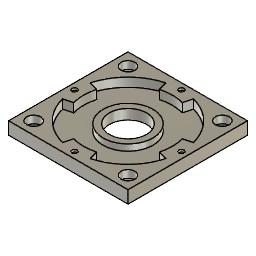
OpenATC-Assembly (Autodesk Fusion 360 archive; units mm, degrees)
design "OpenATC-Base-holder"
Autodesk Fusion 360 part; units mm, degrees
note: some values were not read from the file. Chosen so that the rebuilt part matches the saved one: a direction; a side.
sketch "Sketch1" plane through (0, 0, 0) normal (0, 0, 1) x (1, 0, 0)
  line L0 (-47.5, -47.5) -> (47.5, -47.5)
  line L1 (47.5, -47.5) -> (47.5, 47.5)
  line L2 (47.5, 47.5) -> (-47.5, 47.5)
  line L3 (-47.5, 47.5) -> (-47.5, -47.5)
  line L4 (-37.5, 37.5) -> (-37.5, -37.5) construction
  line L5 (-37.5, -37.5) -> (37.5, -37.5) construction
  line L6 (37.5, 37.5) -> (37.5, -37.5) construction
  line L7 (-37.5, 37.5) -> (-24.7362, 37.5)
  line L8 (-24.7362, 37.5) -> (37.5, 37.5) construction
  line L9 (-47.5, 47.5) -> (47.5, -47.5) construction
  line L10 (-47.5, -47.5) -> (47.5, 47.5) construction
  point P0 (-37.5, 37.5)
  point P1 (37.5, 37.5)
  point P2 (-37.5, -37.5)
  point P3 (37.5, -37.5)
  dimension "d33" = 10
  dimension "d34" = 75
  dimension "d35" = 75
  constraint horizontal L0
  constraint vertical L1
  constraint horizontal L2
  constraint vertical L3
  constraint coincident P0 L4.start
  constraint coincident P2 L4.end
  constraint coincident P3 L5.end
  constraint horizontal L5
  constraint coincident P1 L6.start
  constraint perpendicular L4 L7
  constraint vertical L6
  constraint vertical L4
  constraint horizontal L8
  constraint coincident origin L10
  constraint coincident origin L9
  constraint coincident L0.start L3.end
  constraint coincident P2 L10
  constraint coincident P0 L9
  constraint coincident P1 L10
  measures "d33" distance of L1 L6
  measures "d34" distance of P2 P3
  measures "d35" distance of P0 P2
extrude "Extrude1" add sketch "Sketch1" along normal blind 10
sketch "Sketch2" plane through (0, 0, 10) normal (0, 0, 1) x (-1, 0, 0)
  line L0 (47.5, -47.5) -> (47.5, 47.5)
  line L1 (47.5, 47.5) -> (-47.5, 47.5)
  line L2 (-47.5, 47.5) -> (-47.5, -47.5)
  line L3 (-47.5, -47.5) -> (47.5, -47.5)
  circle A0 centre (0, 0) radius 19.8
  circle A1 centre (0, 0) radius 42.5
  line L4 (0, 0) -> (0, -42.5) construction
  line L5 (10.9998, -41.0518) -> (9.1234, -34.0489)
  line L6 (0, 0) -> (9.1234, -34.0489) construction
  line L7 (0, 0) -> (-9.1234, -34.0489) construction
  line L8 (-9.1234, -34.0489) -> (-10.9998, -41.0518)
  arc A2 (-9.1234, -34.0489) -> (9.1234, -34.0489) centre (0, 0) ccw
  line L9 (41.0518, 10.9998) -> (34.0489, 9.1234)
  arc A3 (34.0489, -9.1234) -> (34.0489, 9.1234) centre (0, 0) ccw
  line L10 (34.0489, -9.1234) -> (41.0518, -10.9998)
  line L11 (-10.9998, 41.0518) -> (-9.1234, 34.0489)
  arc A4 (9.1234, 34.0489) -> (-9.1234, 34.0489) centre (0, 0) ccw
  line L12 (9.1234, 34.0489) -> (10.9998, 41.0518)
  line L13 (-41.0518, -10.9998) -> (-34.0489, -9.1234)
  arc A5 (-34.0489, 9.1234) -> (-34.0489, -9.1234) centre (0, 0) ccw
  line L14 (-34.0489, 9.1234) -> (-41.0518, 10.9998)
  dimension "d9" = 39.6
  dimension "d10" = 85
  dimension "d11" = 35.25
  dimension "d12" = 15
  dimension "d13" = 15
  dimension "d15" = 360
  constraint coincident A0.centre A1.centre
  constraint coincident A1 L4.end
  constraint vertical L4
  constraint coincident A1 L5.start
  constraint coincident A1 L8.end
  constraint parallel L7 L8
  constraint parallel L5 L6
  constraint concentric A1 A2
  measures "d9" diameter of A0
  measures "d10" diameter of A1
  measures "d11" radius of A2
  measures "d12" angle of L4 L5
  measures "d13" angle of L4 L7
extrude "Extrude2" cut sketch "Sketch2" against normal blind 7 contours A1 L5 L8 A2 L9 A3 L10 L11 A4 L12 L13 A5 L14
sketch "Sketch3" plane through (0, 0, 10) normal (0, 0, 1) x (-1, 0, 0)
  circle A0 centre (0, 0) radius 19.8
extrude "Extrude3" cut sketch "Sketch3" against normal up to surface (2 mm away)
sketch "Sketch4" plane through (0, 0, 8) normal (0, 0, 1) x (-1, 0, 0)
  circle A0 centre (0, 0) radius 19.8
  circle A1 centre (0, 0) radius 14.8
  dimension "d36" = 5
  constraint concentric A0 A1
  measures "d36" distance of A0 A1
extrude "Extrude4" cut sketch "Sketch4" against normal through all contours A1
sketch "Sketch6" plane through (0, 0, 10) normal (0, 0, 1) x (-1, 0, 0)
  line L0 (47.5, -47.5) -> (47.5, 47.5)
  line L1 (47.5, 47.5) -> (-47.5, 47.5)
  line L2 (-47.5, 47.5) -> (-47.5, -47.5)
  line L3 (-47.5, -47.5) -> (47.5, -47.5)
  arc A0 (-10.9998, 41.0518) -> (-41.0518, 10.9998) centre (0, 0) ccw
  line L4 (-10.9998, 41.0518) -> (-9.1234, 34.0489)
  arc A1 (9.1234, 34.0489) -> (-9.1234, 34.0489) centre (0, 0) ccw
  line L5 (9.1234, 34.0489) -> (10.9998, 41.0518)
  arc A2 (41.0518, 10.9998) -> (10.9998, 41.0518) centre (0, 0) ccw
  line L6 (41.0518, 10.9998) -> (34.0489, 9.1234)
  arc A3 (34.0489, -9.1234) -> (34.0489, 9.1234) centre (0, 0) ccw
  line L7 (34.0489, -9.1234) -> (41.0518, -10.9998)
  arc A4 (10.9998, -41.0518) -> (41.0518, -10.9998) centre (0, 0) ccw
  line L8 (37.5, -37.5) -> (-37.5, -37.5) construction
  line L9 (-37.5, -37.5) -> (-37.5, 37.5) construction
  line L10 (-37.5, 37.5) -> (37.5, 37.5) construction
  line L11 (37.5, 37.5) -> (37.5, -37.5) construction
  line L12 (-9.1234, -34.0489) -> (-10.9998, -41.0518)
  arc A5 (-41.0518, -10.9998) -> (-10.9998, -41.0518) centre (0, 0) ccw
  line L13 (-41.0518, -10.9998) -> (-34.0489, -9.1234)
  arc A6 (-34.0489, 9.1234) -> (-34.0489, -9.1234) centre (0, 0) ccw
  line L14 (-34.0489, 9.1234) -> (-41.0518, 10.9998)
  line L15 (10.9998, -41.0518) -> (9.1234, -34.0489)
  arc A7 (-9.1234, -34.0489) -> (9.1234, -34.0489) centre (0, 0) ccw
  point P0 (37.5, -37.5)
  point P1 (-37.5, -37.5)
  point P2 (-37.5, 37.5)
  point P3 (37.5, 37.5)
  dimension "d22" = 10
  dimension "d23" = 10
  dimension "d24" = 10
  dimension "d25" = 10
  constraint coincident P0 L8.start
  constraint coincident P1 L8.end
  constraint parallel L3 L8
  constraint coincident P2 L9.end
  constraint perpendicular L3 L9
  constraint coincident P3 L10.end
  constraint perpendicular L9 L10
  constraint vertical L11
  measures "d22" distance of L1 L10
  measures "d23" distance of L0 L11
  measures "d24" distance of L3 L8
  measures "d25" distance of L2 L9
hole "Hole1" at (-37.5, -37.5, 10) at (-37.5, 37.5, 10) at (37.5, 37.5, 10) at (37.5, -37.5, 10) direction (0, 0, -1) diameter 6.6 end through all counterbore diameter 11 counterbore depth 6
sketch "Sketch7" plane through (0, 0, 10) normal (0, 0, 1) x (-1, 0, 0)
  circle A0 centre (-37.5, -37.5) radius 5.5
  circle A1 centre (37.5, 37.5) radius 5.5
  circle A2 centre (37.5, -37.5) radius 5.5
  circle A3 centre (-37.5, 37.5) radius 5.5
  line L0 (47.5, -47.5) -> (47.5, 47.5)
  line L1 (47.5, 47.5) -> (-47.5, 47.5)
  line L2 (-47.5, 47.5) -> (-47.5, -47.5)
  line L3 (-47.5, -47.5) -> (47.5, -47.5)
  line L4 (-9.1234, -34.0489) -> (-10.9998, -41.0518)
  arc A4 (-41.0518, -10.9998) -> (-10.9998, -41.0518) centre (0, 0) ccw
  line L5 (-41.0518, -10.9998) -> (-34.0489, -9.1234)
  arc A5 (-34.0489, 9.1234) -> (-34.0489, -9.1234) centre (0, 0) ccw
  line L6 (-34.0489, 9.1234) -> (-41.0518, 10.9998)
  arc A6 (-10.9998, 41.0518) -> (-41.0518, 10.9998) centre (0, 0) ccw
  line L7 (-10.9998, 41.0518) -> (-9.1234, 34.0489)
  arc A7 (9.1234, 34.0489) -> (-9.1234, 34.0489) centre (0, 0) ccw
  line L8 (9.1234, 34.0489) -> (10.9998, 41.0518)
  arc A8 (41.0518, 10.9998) -> (10.9998, 41.0518) centre (0, 0) ccw
  line L9 (41.0518, 10.9998) -> (34.0489, 9.1234)
  arc A9 (34.0489, -9.1234) -> (34.0489, 9.1234) centre (0, 0) ccw
  line L10 (34.0489, -9.1234) -> (41.0518, -10.9998)
  arc A10 (10.9998, -41.0518) -> (41.0518, -10.9998) centre (0, 0) ccw
  line L11 (10.9998, -41.0518) -> (9.1234, -34.0489)
  arc A11 (-9.1234, -34.0489) -> (9.1234, -34.0489) centre (0, 0) ccw
  line L12 (47.5, 0) -> (-47.5, 0) construction
  line L13 (0, -47.5) -> (0, 47.5) construction
  point P0 (42.5, 0)
  point P1 (-42.5, 0)
  point P2 (0, -42.5)
  point P3 (0, 42.5)
  dimension "d37" = 5
  dimension "d38" = 5
  dimension "d39" = 5
  dimension "d40" = 5
  constraint midpoint L0 L12.start
  constraint midpoint L2 L12.end
  constraint midpoint L3 L13.start
  constraint midpoint L1 L13.end
  constraint coincident L12 P0
  constraint coincident L12 P1
  constraint coincident L13 P2
  constraint coincident L13 P3
  measures "d37" distance of L0 P0
  measures "d38" distance of L1 P3
  measures "d39" distance of L2 P1
  measures "d40" distance of L3 P2
hole "Hole2" at (0, 42.5, 10) at (-42.5, 0, 10) at (0, -42.5, 10) at (42.5, 0, 10) direction (0, 0, -1) diameter 3.332 end through all
thread "Thread1" "ISO Metric profile 4.0 M4x0.7 M4x0.7 6H" thread offset 0 thread depth 7.4
chamfer "Chamfer1" distance 0.4 angle 75 4 edges at (-1.5533, 43.1025, 10) (40.9467, 0.6025, 10) (-1.5533, -41.8975, 10) (-44.0533, 0.6025, 10) measured on face at (-5.2099, -39.359, 10) measured on face at (-5.2099, -39.359, 10) measured on face at (-5.2099, -39.359, 10) measured on face at (-5.2099, -39.359, 10)
equation "d13 = d12"
equation "d23 = d22"
equation "d24 = d22"
equation "d25 = d22"
equation "d35 = d34"
equation "d38 = d37"
equation "d39 = d37"
equation "d40 = d37"

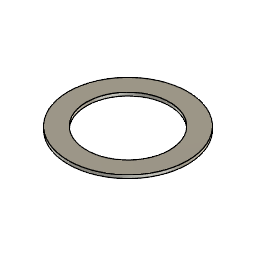
design "Washer-ID_25mm-OD_36mm"
Autodesk Fusion 360 part; units mm, degrees
sketch "Sketch1" plane through (0, 0, 0) normal (0, 0, 1) x (1, 0, 0)
  circle A0 centre (0, 0) radius 12.5
  circle A1 centre (0, 0) radius 18
  dimension "d1" = 25
  dimension "d2" = 36
  constraint coincident A0.centre A1.centre
  constraint concentric A0 A1
  measures "d1" diameter of A0
  measures "d2" diameter of A1
extrude "Extrude1" add sketch "Sketch1" along normal blind 1

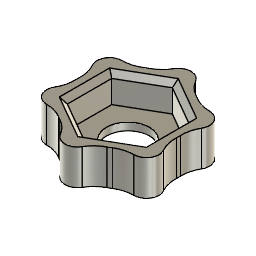
design "OpenATC-ER20-A-Nut-holder"
Autodesk Fusion 360 part; units mm, degrees
sketch "Sketch1" plane through (0, 0, 0) normal (0, 0, 1) x (1, 0, 0)
  circle A0 centre (0, 0) radius 8.5
  circle A1 centre (0, 0) radius 20
  dimension "d1" = 17
  dimension "d2" = 40
  constraint coincident A0.centre A1.centre
  measures "d1" diameter of A0
  measures "d2" diameter of A1
extrude "Extrude1" add sketch "Sketch1" along normal blind 14
sketch "Sketch2" plane through (0, 0, 14) normal (0, 0, 1) x (-1, 0, 0)
  circle A0 centre (0, 0) radius 8.5
  circle A1 centre (0, 0) radius 20
  line L0 (-15.25, -8.8046) -> (0, -17.6092)
  line L1 (0, -17.6092) -> (15.25, -8.8046)
  line L2 (15.25, -8.8046) -> (15.25, 8.8046)
  line L3 (15.25, 8.8046) -> (0, 17.6092)
  line L4 (0, 17.6092) -> (-15.25, 8.8046)
  line L5 (-15.25, 8.8046) -> (-15.25, -8.8046)
  line L6 (0, 0) -> (0, -24.7489) construction
  dimension "d5" = 15.25
  constraint coincident A0.centre A1.centre
  constraint vertical L6
  constraint coincident L0.end L6
  measures "d5" distance of A0.centre L5
extrude "Extrude2" cut sketch "Sketch2" against normal blind 11 contours L0 L1 L2 L3 L4 L5
sketch "Sketch3" plane through (0, 0, 14) normal (0, 0, 1) x (-1, 0, 0)
  line L0 (0, -17.6092) -> (-15.25, -8.8046)
  line L1 (-15.25, -8.8046) -> (-15.25, 8.8046)
  line L2 (-15.25, 8.8046) -> (0, 17.6092)
  line L3 (0, 17.6092) -> (15.25, 8.8046)
  line L4 (15.25, 8.8046) -> (15.25, -8.8046)
  line L5 (15.25, -8.8046) -> (0, -17.6092)
  circle A0 centre (0, 0) radius 20
  line L6 (0, -20) -> (0, 20) construction
  line L7 (20, 0) -> (-20, 0) construction
  arc A1 (-4.3301, -22.5) -> (4.3301, -22.5) centre (0, -20) ccw
  line L8 (0, -20) -> (0, -25) construction
  line L9 (0, -20) -> (4.3301, -22.5) construction
  line L10 (0, -20) -> (-4.3301, -22.5) construction
  arc A2 (9.3264, -17.6923) -> (4.3301, -22.5) centre (15.1554, -28.75) ccw
  arc A3 (-4.3301, -22.5) -> (-9.3264, -17.6923) centre (-15.1554, -28.75) ccw
  arc A4 (-9.3264, -17.6923) -> (9.3264, -17.6923) centre (0, 0) ccw
  arc A5 (17.3205, -15) -> (21.6506, -7.5) centre (17.3205, -10) ccw
  arc A6 (17.3205, -15) -> (10.6588, -16.9231) centre (17.3205, -27.5) ccw
  arc A7 (10.6588, -16.9231) -> (19.9852, -0.7692) centre (0, 0) ccw
  arc A8 (19.9852, -0.7692) -> (21.6506, -7.5) centre (32.476, -1.25) ccw
  arc A9 (21.6506, 7.5) -> (17.3205, 15) centre (17.3205, 10) ccw
  arc A10 (21.6506, 7.5) -> (19.9852, 0.7692) centre (32.476, 1.25) ccw
  arc A11 (19.9852, 0.7692) -> (10.6588, 16.9231) centre (0, 0) ccw
  arc A12 (10.6588, 16.9231) -> (17.3205, 15) centre (17.3205, 27.5) ccw
  arc A13 (4.3301, 22.5) -> (-4.3301, 22.5) centre (0, 20) ccw
  arc A14 (4.3301, 22.5) -> (9.3264, 17.6923) centre (15.1554, 28.75) ccw
  arc A15 (9.3264, 17.6923) -> (-9.3264, 17.6923) centre (0, 0) ccw
  arc A16 (-9.3264, 17.6923) -> (-4.3301, 22.5) centre (-15.1554, 28.75) ccw
  arc A17 (-17.3205, 15) -> (-21.6506, 7.5) centre (-17.3205, 10) ccw
  arc A18 (-17.3205, 15) -> (-10.6588, 16.9231) centre (-17.3205, 27.5) ccw
  arc A19 (-10.6588, 16.9231) -> (-19.9852, 0.7692) centre (0, 0) ccw
  arc A20 (-19.9852, 0.7692) -> (-21.6506, 7.5) centre (-32.476, 1.25) ccw
  arc A21 (-21.6506, -7.5) -> (-17.3205, -15) centre (-17.3205, -10) ccw
  arc A22 (-21.6506, -7.5) -> (-19.9852, -0.7692) centre (-32.476, -1.25) ccw
  arc A23 (-19.9852, -0.7692) -> (-10.6588, -16.9231) centre (0, 0) ccw
  arc A24 (-10.6588, -16.9231) -> (-17.3205, -15) centre (-17.3205, -27.5) ccw
  dimension "d10" = 60
  dimension "d11" = 60
  dimension "d12" = 5
  dimension "d14" = 360
  constraint coincident A0 L6.start
  constraint coincident A0 L6.end
  constraint vertical L6
  constraint coincident A0 L7.start
  constraint coincident A0 L7.end
  constraint perpendicular L6 L7
  constraint coincident A0.centre L6
  constraint coincident A0.centre L7
  constraint parallel L6 L8
  constraint coincident L6.start A1.centre
  constraint tangent A0 A2
  constraint coincident A0 A2.start
  constraint tangent A1 A2
  constraint tangent A0 A3
  constraint coincident A0 A3.end
  constraint tangent A1 A3
  constraint coincident A1 L8.end
  constraint coincident L6.start A4
  measures "d10" angle of L8 L10
  measures "d11" angle of L8 L9
  measures "d12" radius of A1
extrude "Extrude3" add sketch "Sketch3" against normal up to surface (14 mm away) contours A0 A9 A10 A11 A12 | A0 A5 A6 A7 A8 | A0 A13 A14 A15 A16 | A0 A1 A2 A3 A4 | A0 A17 A18 A19 A20 | A0 A21 A22 A23 A24
chamfer "Chamfer1" distance 2 angle 45 6 edges at (-7.625, 13.2069, 14) (-15.25, 0, 14) (-7.625, -13.2069, 14) (7.625, -13.2069, 14) (15.25, 0, 14) (7.625, 13.2069, 14)
sketch "Sketch4" plane through (0, 0, 0) normal (0, 0, -1) x (1, 0, 0)
  circle A0 centre (0, 0) radius 8.5
  arc A1 (-9.3264, 17.6923) -> (-10.6588, 16.9231) centre (0, 0) ccw
  arc A2 (-17.3205, 15) -> (-10.6588, 16.9231) centre (-17.3205, 27.5) ccw
  arc A3 (-17.3205, 15) -> (-21.6506, 7.5) centre (-17.3205, 10) ccw
  arc A4 (-19.9852, 0.7692) -> (-21.6506, 7.5) centre (-32.476, 1.25) ccw
  arc A5 (-19.9852, 0.7692) -> (-19.9852, -0.7692) centre (0, 0) ccw
  arc A6 (-21.6506, -7.5) -> (-19.9852, -0.7692) centre (-32.476, -1.25) ccw
  arc A7 (-21.6506, -7.5) -> (-17.3205, -15) centre (-17.3205, -10) ccw
  arc A8 (-10.6588, -16.9231) -> (-17.3205, -15) centre (-17.3205, -27.5) ccw
  arc A9 (-10.6588, -16.9231) -> (-9.3264, -17.6923) centre (0, 0) ccw
  arc A10 (-4.3301, -22.5) -> (-9.3264, -17.6923) centre (-15.1554, -28.75) ccw
  arc A11 (-4.3301, -22.5) -> (4.3301, -22.5) centre (0, -20) ccw
  arc A12 (9.3264, -17.6923) -> (4.3301, -22.5) centre (15.1554, -28.75) ccw
  arc A13 (9.3264, -17.6923) -> (10.6588, -16.9231) centre (0, 0) ccw
  arc A14 (17.3205, -15) -> (10.6588, -16.9231) centre (17.3205, -27.5) ccw
  arc A15 (17.3205, -15) -> (21.6506, -7.5) centre (17.3205, -10) ccw
  arc A16 (19.9852, -0.7692) -> (21.6506, -7.5) centre (32.476, -1.25) ccw
  arc A17 (19.9852, -0.7692) -> (19.9852, 0.7692) centre (0, 0) ccw
  arc A18 (21.6506, 7.5) -> (19.9852, 0.7692) centre (32.476, 1.25) ccw
  arc A19 (21.6506, 7.5) -> (17.3205, 15) centre (17.3205, 10) ccw
  arc A20 (10.6588, 16.9231) -> (17.3205, 15) centre (17.3205, 27.5) ccw
  arc A21 (10.6588, 16.9231) -> (9.3264, 17.6923) centre (0, 0) ccw
  arc A22 (4.3301, 22.5) -> (9.3264, 17.6923) centre (15.1554, 28.75) ccw
  arc A23 (4.3301, 22.5) -> (-4.3301, 22.5) centre (0, 20) ccw
  arc A24 (-9.3264, 17.6923) -> (-4.3301, 22.5) centre (-15.1554, 28.75) ccw
  circle A25 centre (0, 0) radius 13.25
  circle A26 centre (0, 0) radius 15.75
  dimension "d18" = 26.5
  dimension "d19" = 31.5
  constraint coincident A0.centre A1.centre
  constraint concentric A0 A26
  measures "d18" diameter of A25
  measures "d19" diameter of A26
extrude "Extrude4" cut sketch "Sketch4" against normal blind 1 contours A26
equation "d11 = d10"

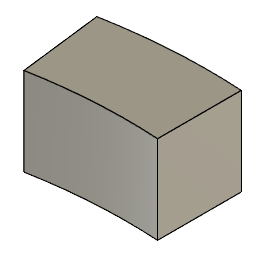
design "OpenATC-shock-absorber"
Autodesk Fusion 360 part; units mm, degrees
sketch "Sketch1" plane through (0, 0, 0) normal (0, 0, 1) x (1, 0, 0)
  line L0 (0, 0) -> (-9.0099, 73.3797)
  line L1 (0, 0) -> (0, 8.9683)
  line L2 (0, 8.9683) -> (0, 73.9307)
  line L3 (-9.0099, 73.3797) -> (-9.7404, 79.3294)
  line L4 (0, 73.9307) -> (0, 79.9251)
  arc A0 (0, 73.9307) -> (-9.0099, 73.3797) centre (-2.263, 37) ccw
  arc A1 (0, 79.9251) -> (-9.7404, 79.3294) centre (-2.4465, 40) ccw
  line L5 (0, 0) -> (0, 2.8792)
  line L6 (0, 0) -> (-8.5021, 139.0084) construction
  dimension "d1" = 37
  dimension "d2" = 40
  dimension "d4" = 3.5
  dimension "d5" = 37
  dimension "d6" = 40
  dimension "d7" = 3.5
  constraint coincident L0.start L1.start
  constraint vertical L1
  constraint parallel L1 L2
  constraint parallel L0 L3
  constraint parallel L2 L4
  constraint coincident L1 L5.end
  constraint coincident A1.centre L6
  constraint coincident A0.centre L6
  measures "d1" radius of A0
  measures "d2" radius of A1
  measures "d4" angle of L4 L6
  measures "d5" vertical distance of L0.start A0.centre
  measures "d6" vertical distance of L0.start A1.centre
  measures "d7" angle of L0 L6
extrude "Extrude1" add sketch "Sketch1" along normal blind 6.3 contours L3 L4 A0 A1
equation "d5 = d1"
equation "d6 = d2"
equation "d7 = d4"

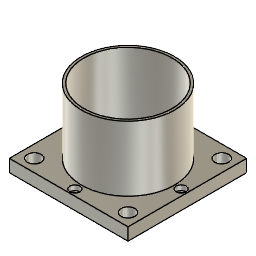
design "OpenATC-Base-bottom-cover"
Autodesk Fusion 360 part; units mm, degrees
sketch "Sketch1" plane through (0, 0, 0) normal (0, 0, 1) x (1, 0, 0)
  line L0 (-47.5, 47.5) -> (47.5, 47.5)
  line L1 (47.5, 47.5) -> (47.5, -47.5)
  line L2 (47.5, -47.5) -> (-47.5, -47.5)
  line L3 (-47.5, -47.5) -> (-47.5, 47.5)
  line L4 (-47.5, 47.5) -> (47.5, -47.5) construction
  line L5 (-47.5, -47.5) -> (47.5, 47.5) construction
  circle A0 centre (0, 0) radius 35.2
  dimension "d1" = 95
  dimension "d2" = 95
  dimension "d3" = 70.4
  constraint horizontal L0
  constraint vertical L1
  constraint horizontal L2
  constraint vertical L3
  constraint coincident A0.centre L4
  constraint coincident A0.centre L5
  constraint coincident A0.centre origin
  measures "d1" distance of L1.end L2.end
  measures "d2" distance of L0.start L2.end
  measures "d3" diameter of A0
extrude "Extrude1" add sketch "Sketch1" along normal blind 10
sketch "Sketch2" plane through (0, 0, 10) normal (0, 0, 1) x (-1, 0, 0)
  circle A0 centre (0, 0) radius 35.2
  line L0 (47.5, 47.5) -> (-47.5, 47.5)
  line L1 (-47.5, 47.5) -> (-47.5, -47.5)
  line L2 (-47.5, -47.5) -> (47.5, -47.5)
  line L3 (47.5, -47.5) -> (47.5, 47.5)
  line L4 (42.5, 0) -> (-42.5, 0) construction
  line L5 (0, -42.5) -> (0, 42.5) construction
  point P0 (0, -42.5)
  point P1 (42.5, 0)
  point P2 (0, 42.5)
  point P3 (-42.5, 0)
  dimension "d7" = 5
  dimension "d8" = 5
  dimension "d9" = 5
  dimension "d10" = 5
  constraint coincident P1 L4.start
  constraint coincident P3 L4.end
  constraint coincident P0 L5.start
  constraint coincident P2 L5.end
  constraint perpendicular L0 L5
  constraint horizontal L4
  constraint coincident A0.centre L4
  constraint coincident A0.centre L5
  measures "d7" distance of L0 P2
  measures "d8" distance of L3 P1
  measures "d9" distance of L1 P3
  measures "d10" distance of L2 P0
hole "Hole1" at (-42.5, 0, 10) at (0, 42.5, 10) at (42.5, 0, 10) at (0, -42.5, 10) direction (0, 0, -1) diameter 4.5 depth 15 tip angle 118 counterbore diameter 8 counterbore depth 4
sketch "Sketch3" plane through (0, 0, 10) normal (0, 0, 1) x (-1, 0, 0)
  circle A0 centre (-42.5, 0) radius 4
  circle A1 centre (42.5, 0) radius 4
  circle A2 centre (0, -42.5) radius 4
  circle A3 centre (0, 42.5) radius 4
  circle A4 centre (0, 0) radius 35.2
  line L0 (47.5, 47.5) -> (-47.5, 47.5)
  line L1 (-47.5, 47.5) -> (-47.5, -47.5)
  line L2 (-47.5, -47.5) -> (47.5, -47.5)
  line L3 (47.5, -47.5) -> (47.5, 47.5)
  circle A5 centre (0, 0) radius 35.2
  circle A6 centre (0, 0) radius 37.2
  dimension "d16" = 2
  constraint concentric A4 A5
  constraint concentric A5 A6
  constraint tangent A4 A5
  measures "d16" distance of A5 A6
extrude "Extrude2" add sketch "Sketch3" along normal blind 52 contours A6
sketch "Sketch4" plane through (0, 0, 10) normal (0, 0, 1) x (-1, 0, 0)
  circle A0 centre (0, 0) radius 37.2
  circle A1 centre (-42.5, 0) radius 4
  circle A2 centre (42.5, 0) radius 4
  circle A3 centre (0, -42.5) radius 4
  circle A4 centre (0, 42.5) radius 4
  line L0 (47.5, 47.5) -> (-47.5, 47.5)
  line L1 (-47.5, 47.5) -> (-47.5, -47.5)
  line L2 (-47.5, -47.5) -> (47.5, -47.5)
  line L3 (47.5, -47.5) -> (47.5, 47.5)
  line L4 (37.5, -37.5) -> (-37.5, -37.5) construction
  line L5 (-37.5, -37.5) -> (-37.5, 37.5) construction
  line L6 (-37.5, 37.5) -> (37.5, 37.5) construction
  line L7 (37.5, 37.5) -> (37.5, -37.5) construction
  point P0 (37.5, -37.5)
  point P1 (-37.5, -37.5)
  point P2 (-37.5, 37.5)
  point P3 (37.5, 37.5)
  dimension "d19" = 10
  dimension "d20" = 10
  dimension "d21" = 10
  dimension "d22" = 10
  constraint horizontal L4
  constraint vertical L5
  constraint horizontal L6
  constraint vertical L7
  constraint coincident P0 L4.start
  constraint coincident P1 L4.end
  constraint coincident P2 L5.end
  constraint coincident P3 L6.end
  measures "d19" distance of L0 L6
  measures "d20" distance of L3 L7
  measures "d21" distance of L2 L4
  measures "d22" distance of L1 L5
hole "Hole2" at (-37.5, -37.5, 10) at (-37.5, 37.5, 10) at (37.5, 37.5, 10) at (37.5, -37.5, 10) direction (0, 0, -1) diameter 11 end through all
equation "d2 = d1"
equation "d8 = d7"
equation "d9 = d7"
equation "d10 = d7"
equation "d20 = d19"
equation "d21 = d19"
equation "d22 = d19"
